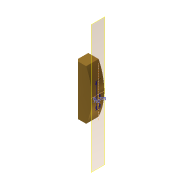
# Autodesk Inventor part: Radial Bushing
Saved by Autodesk Inventor 2014 SP1 (Build 180222100, 222)
## iProperties
Created: 2014-04-22
Part Number: Radial Bushing
Material: Generic
Document SubType Name: Modeling
Designer: Rauhul Varma
Density: 1 g/cm^3
Appearance: Brass - Satin
Author: Rauhul Varma
Autodesk Inventor part; units mm, degrees
ref_plane "XZ Plane" through (0, 0, 0) normal (0, 1, 0) x (-1, 0, 0)
ref_plane "XY Plane" through (0, 0, 0) normal (0, 0, 1) x (1, 0, 0)
sketch "Sketch1" plane through (0, 0, 0) normal (0, 0, 1) x (1, 0, 0)
  circle A0 centre (0, 0) radius 44.45
  line L0 (-32.2263, -21.7487) -> (32.2263, -21.7487) construction
  line L1 (32.2263, -21.7487) -> (32.2263, 21.7487)
  line L2 (32.2263, 21.7487) -> (-32.2263, 21.7487) construction
  line L3 (-32.2263, 21.7487) -> (-32.2263, -21.7487) construction
  line L4 (-32.2263, -21.7487) -> (32.2263, 21.7487) construction
  line L5 (32.2263, -21.7487) -> (-32.2263, 21.7487) construction
  line L6 (-23.8125, -30.1625) -> (23.8125, -30.1625) construction
  line L7 (23.8125, -30.1625) -> (23.8125, 30.1625) construction
  line L8 (23.8125, 30.1625) -> (-23.8125, 30.1625) construction
  line L9 (-23.8125, 30.1625) -> (-23.8125, -30.1625) construction
  line L10 (-23.8125, -30.1625) -> (23.8125, 30.1625) construction
  line L11 (23.8125, -30.1625) -> (-23.8125, 30.1625) construction
  line L12 (-32.2263, 21.7487) -> (-23.8125, 30.1625) construction
  line L13 (-32.2263, -21.7487) -> (-23.8125, -30.1625) construction
  line L14 (23.8125, -30.1625) -> (32.2263, -21.7487) construction
  line L15 (32.2263, 21.7487) -> (23.8125, 30.1625) construction
  line L16 (32.2263, 0) -> (44.45, 0) construction
  line L17 (40.1609, 19.05) -> (32.2263, 19.05)
  line L18 (32.2263, -19.05) -> (40.1609, -19.05)
  dimension "d0" = 88.9
  dimension "d2" = 64.4525
  dimension "d5" = 47.625
  dimension "d6" = 60.325
  dimension "d18" = 45
  dimension "d22" = 19.05
  dimension "d23" = 19.05
  constraints: 38 end point, 6 parallel, 5 midpoint, 4 perpendicular, 3 point on circle, 2 horizontal, 2 point on line, 1 centre point, 1 coincident
  measures "d0" diameter of A0
  measures "d2" distance of L1.end L2.end
  measures "d5" distance of L8.end L7.end
  measures "d6" distance of L8.end L6.start
  measures "d18" angle of L12 L2
  measures "d22" distance between parallel lines of L16 L17
  measures "d23" distance between parallel lines of L18 L16
extrude "Extrusion1" add sketch "Sketch1" along normal blind 9.525 contours A0 L18 L1 L17 picked at (36.3009, 0)
ref_plane "Work Plane1" through (44.45, 0, 0) normal (1, 0, 0) x (0, 1, 0)
sketch "Sketch2" plane through (44.45, 0, 0) normal (1, 0, 0) x (0, 1, 0)
  line L0 (0, 9.9848) -> (0, 0) construction
  line L1 (-19.05, 4.7625) -> (19.05, 4.7625) construction
  line L2 (19.05, 0) -> (-19.05, 0) projected
  line L3 (-19.05, 0) -> (-19.05, 9.525) projected
  line L4 (19.05, 9.525) -> (-19.05, 9.525) projected
  line L5 (19.05, 0) -> (19.05, 9.525) projected
  point P0 (-9.525, 4.7625)
  point P1 (9.525, 4.7625)
  dimension "d9" = 19.05
  dimension "d10" = 9.525
  constraints: 4 end point, 2 midpoint, 2 point on line, 1 perpendicular, 1 vertical
  measures "d9" distance of point (-9.525, 4.762) point (9.525, 4.762)
  measures "d10" distance from line of L0 point (-9.525, 4.762)
hole "Hole2" at (44.45, -9.525, 4.7625) at (44.45, 9.525, 4.7625) direction (-1, 0, 0) diameter 3.6576 end through all counterbore diameter 6.858 counterbore depth 4.445 clearance for "Socket Head Cap Screw" size "#6" standard "Ansi Unified Screw Threads"
equation "\"d10\" = 0.5 * d9"
body "Solid1"
